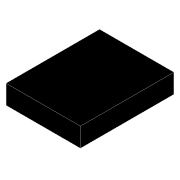
# Autodesk Inventor part: SCANLAB-SNZ0045937
Saved by Autodesk Inventor 2022 (Build 260153000, 153)
## iProperties
Created: 2024-04-12
Part Number: SCANLAB-SNZ0045937
Material: Generic
Document SubType Name: Modeling
Designer: LaptopJR
Density: 1 g/cm^3
Appearance: Anodized - Black
Author: LaptopJR
Autodesk Inventor part; units mm, degrees
ref_plane "YZ Plane" through (0, 0, 0) normal (1, 0, 0) x (0, 1, 0)
ref_plane "XZ Plane" through (0, 0, 0) normal (0, 1, 0) x (-1, 0, 0)
ref_plane "XY Plane" through (0, 0, 0) normal (0, 0, 1) x (1, 0, 0)
sketch "Sketch1" plane through (0, 0, 0) normal (0, 1, 0) x (-1, 0, 0)
  line L0 (0, 0) -> (-175, 0)
  line L1 (-175, 0) -> (-175, -220)
  line L2 (-175, -220) -> (0, -220)
  line L3 (0, -220) -> (0, 0)
  dimension "d0" = 175
  dimension "d1" = 220
  constraints: 8 end point, 2 parallel, 1 horizontal, 1 perpendicular
  measures "d0" distance of L1.end L2.end
  measures "d1" distance of L0.end L1.end
extrude "Extrusion1" add sketch "Sketch1" along normal blind 45
sketch "Sketch2" plane through (0, 0, 0) normal (0, -1, 0) x (1, 0, 0)
  line L0 (175, 0) -> (175, -220) construction
  line L1 (175, -110) -> (0, -110) construction
  line L2 (0, -220) -> (0, 0) projected
  line L3 (16.1074, -21.1997) -> (158.8926, -21.1997) construction
  line L4 (158.8926, -21.1997) -> (158.8926, -198.8003) construction
  line L5 (158.8926, -198.8003) -> (16.1074, -198.8003) construction
  line L6 (16.1074, -198.8003) -> (16.1074, -21.1997) construction
  line L7 (16.1074, -21.1997) -> (158.8926, -198.8003) construction
  line L8 (158.8926, -21.1997) -> (16.1074, -198.8003) construction
  circle A0 centre (158.8926, -21.1997) radius 5
  circle A1 centre (158.8926, -198.8003) radius 5
  circle A2 centre (16.1074, -198.8003) radius 5
  circle A3 centre (16.1074, -21.1997) radius 5
  point P0 (87.5, -110)
  dimension "d4" = 10
  constraints: 14 end point, 5 midpoint, 4 centre point, 4 coincident, 3 equal radius, 2 parallel, 1 horizontal, 1 perpendicular
  measures "d4" diameter of A1
extrude "Extrusion2" add sketch "Sketch2" along normal blind 5
body "Solid1"
